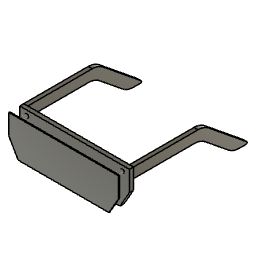
HyperShades mk.1 (Autodesk Fusion 360 design; units mm, degrees)
Autodesk Fusion 360 part; units mm, degrees
sketch "Sketch1" plane through (0, 0, 0) normal (0, 1, 0) x (1, 0, 0)
  line L0 (-69.215, 0) -> (69.215, 0)
  line L1 (-69.215, 0) -> (-69.215, 25.4)
  line L2 (69.215, 0) -> (69.215, 25.4)
  line L3 (69.215, 25.4) -> (57.1899, 46.228)
  line L4 (57.1899, 46.228) -> (-0.1294, 46.228)
  line L5 (-69.215, 25.4) -> (-57.1899, 46.228)
  line L6 (-57.1899, 46.228) -> (-0.1294, 46.228)
  dimension "d1" = 138.43
  dimension "d3" = 25.4
  dimension "d4" = 25.4
  dimension "d5" = 150
  dimension "d6" = 150
  dimension "d26" = 46.228
  constraint horizontal L0
  constraint coincident origin L0
  constraint perpendicular L0 L1
  constraint perpendicular L0 L2
  constraint coincident L0 origin
  constraint midpoint L0 origin
  constraint horizontal L4
  constraint horizontal L6
  measures "d1" distance of L0.start L0.end
  measures "d3" distance of L0.start L1.end
  measures "d4" distance of L0.end L2.end
  measures "d5" angle of L2 L3
  measures "d6" angle of L1 L5
  measures "d26" vertical distance of origin L4.end
extrude "Extrude1" add sketch "Sketch1" along normal blind 1.27 makes body 1
sketch "Sketch2" plane through (0, 1.27, 0) normal (0, 1, 0) x (-1, 0, 0)
  line L0 (69.215, 0) -> (-69.215, 0)
  line L1 (-69.215, 0) -> (-69.215, -25.4)
  line L2 (-69.215, -25.4) -> (-57.1899, -46.228)
  line L3 (-57.1899, -46.228) -> (57.1899, -46.228)
  line L4 (57.1899, -46.228) -> (69.215, -25.4)
  line L5 (69.215, -25.4) -> (69.215, 0)
  circle A0 centre (-60.325, -6.35) radius 2.286
  line L6 (-69.215, 0) -> (-60.325, 0) construction
  line L7 (-60.325, 0) -> (-60.325, -6.35) construction
  line L8 (-60.325, -6.35) -> (-69.215, -6.35) construction
  line L9 (-69.215, -6.35) -> (-69.215, 0) construction
  line L10 (69.215, 0) -> (60.325, 0) construction
  line L11 (60.325, 0) -> (60.325, -6.35) construction
  line L12 (60.325, -6.35) -> (69.215, -6.35) construction
  line L13 (69.215, -6.35) -> (69.215, 0) construction
  circle A1 centre (60.325, -6.35) radius 2.286
  line L14 (0, -46.228) -> (-12.7, -46.228) construction
  line L15 (-12.7, -46.228) -> (-12.7, -30.988) construction
  line L16 (-12.7, -30.988) -> (0, -30.988) construction
  line L17 (0, -30.988) -> (0, -46.228) construction
  line L18 (0, -46.228) -> (12.7, -46.228) construction
  line L19 (12.7, -46.228) -> (12.7, -30.988) construction
  line L20 (12.7, -30.988) -> (0, -30.988) construction
  line L21 (0, -30.988) -> (0, -46.228) construction
  circle A2 centre (-12.7, -30.988) radius 2.286
  circle A3 centre (12.7, -30.988) radius 2.286
  dimension "d10" = 4.572
  dimension "d11" = 8.89
  dimension "d12" = 6.35
  dimension "d23" = 8.89
  dimension "d24" = 6.35
  dimension "d25" = 4.572
  dimension "d27" = 12.7
  dimension "d28" = 15.24
  dimension "d29" = 12.7
  dimension "d30" = 15.24
  dimension "d31" = 4.572
  dimension "d32" = 4.572
  constraint horizontal L6
  constraint vertical L7
  constraint horizontal L8
  constraint vertical L9
  constraint coincident L0.end L1.start
  constraint coincident A0.centre L7.end
  constraint horizontal L10
  constraint vertical L11
  constraint horizontal L12
  constraint vertical L13
  constraint coincident L0.start L5.end
  constraint coincident L11.end L12.start
  constraint horizontal L14
  constraint vertical L15
  constraint horizontal L16
  constraint vertical L17
  constraint midpoint L3 L14.start
  constraint horizontal L18
  constraint vertical L19
  constraint horizontal L20
  constraint vertical L21
  constraint coincident L15.end L16.start
  constraint coincident L19.end L20.start
  measures "d10" diameter of A0
  measures "d11" distance of L0.end L6.end
  measures "d12" distance of L0.end L8.end
  measures "d23" distance of L0.start L10.end
  measures "d24" distance of L0.start L12.end
  measures "d25" diameter of A1
  measures "d27" distance of L14.start L14.end
  measures "d28" distance of L14.start L16.end
  measures "d29" distance of L14.start L18.end
  measures "d30" distance of L14.start L16.end
  measures "d31" diameter of A2
  measures "d32" diameter of A3
extrude "Extrude2" add sketch "Sketch2" along normal blind 12.7 separate body contours A0 | A1 | A2 | A3 makes body 2 at (58.0504, 9.7367, -6.5776) makes body 3 at (-62.5996, 9.7367, -6.5776) makes body 4 at (10.4254, 9.7367, -31.2156) makes body 5 at (-14.9746, 9.7367, -31.2156)
sketch "Sketch3" plane through (0, 13.97, 0) normal (0, 1, 0) x (-1, 0, 0)
  circle A0 centre (-60.325, -6.35) radius 2.286
  line L0 (69.215, 0) -> (-69.215, 0)
  line L1 (-69.215, 0) -> (-69.215, -25.4)
  line L2 (-69.215, -25.4) -> (-57.1899, -46.228)
  line L3 (-57.1899, -46.228) -> (57.1899, -46.228)
  line L4 (57.1899, -46.228) -> (69.215, -25.4)
  line L5 (69.215, -25.4) -> (69.215, 0)
  line L6 (-12.7, -46.228) -> (12.7, -46.228)
  line L7 (-12.7, -46.228) -> (-3.556, -22.4537)
  line L8 (3.556, -22.4537) -> (12.7, -46.228)
  arc A1 (3.556, -22.4537) -> (-3.556, -22.4537) centre (0, -23.8214) ccw
  circle A2 centre (-12.7, -30.988) radius 2.286
  circle A3 centre (12.7, -30.988) radius 2.286
  circle A4 centre (60.325, -6.35) radius 2.286
  point P0 (0, -46.228)
  point P1 (0, -13.208)
  dimension "d15" = 25.4
  dimension "d17" = 33.02
  dimension "d20" = 3.81
  constraint coincident L3 L6.start
  constraint parallel L3 L6
  constraint coincident L6 P0
  constraint midpoint L6 P0
  constraint vertical origin P0
  constraint vertical origin P1
  constraint coincident P1 L8
  constraint coincident P1 L7
  constraint tangent L8 A1
  constraint tangent L7 A1
  measures "d15" distance of L6.start L6.end
  measures "d17" vertical distance of L6.end P1
  measures "d20" radius of A1
extrude "Extrude4" add sketch "Sketch3" along normal blind 5.08 separate body contours L0 L1 L2 L3 L4 L5 L7 L8 A1 makes body 6
sketch "Sketch4" plane through (69.215, 0, 0) normal (1, 0, 0) x (0, 1, 0)
  line L0 (13.97, 0) -> (13.97, -25.4)
  line L1 (13.97, -25.4) -> (19.05, -25.4)
  line L2 (19.05, -25.4) -> (19.05, 0)
  line L3 (19.05, 0) -> (13.97, 0)
  line L4 (19.05, 0) -> (161.29, 0) construction
  line L5 (19.05, 0) -> (100.287, 0)
  line L6 (113.8983, -4.8311) -> (162.0907, -43.9722)
  line L7 (19.05, -12.7) -> (95.7793, -12.7)
  line L8 (109.3906, -17.5311) -> (138.7753, -41.3969)
  line L9 (152.3866, -46.228) -> (161.29, -46.228)
  arc A0 (138.7753, -41.3969) -> (152.3866, -46.228) centre (152.3866, -24.638) ccw
  arc A1 (161.29, -46.228) -> (162.0907, -43.9722) centre (161.29, -44.958) ccw
  arc A2 (109.3906, -17.5311) -> (95.7793, -12.7) centre (95.7793, -34.29) ccw
  arc A3 (113.8983, -4.8311) -> (100.287, 0) centre (100.287, -21.59) ccw
  point P0 (107.95, 0)
  point P1 (19.05, -46.228)
  dimension "d33" = 142.24
  dimension "d34" = 88.9
  dimension "d36" = 12.7
  dimension "d39" = 21.59
  dimension "d40" = 1.27
  dimension "d41" = 21.59
  dimension "d42" = 21.59
  constraint coincident L2.end L3.start
  constraint perpendicular L2 L4
  constraint perpendicular L2 L5
  constraint midpoint L2 L7.start
  constraint perpendicular L2 L7
  constraint parallel L6 L8
  constraint parallel L7 L9
  constraint tangent L8 A0
  constraint tangent L9 A0
  constraint tangent L6 A1
  constraint tangent L9 A1
  constraint tangent L7 A2
  constraint tangent L8 A2
  constraint coincident P0 L5
  constraint coincident P0 L6
  constraint tangent L5 A3
  constraint tangent L6 A3
  constraint horizontal P1 L9.start
  constraint vertical L4.end A1.centre
  measures "d33" distance of L2.end L4.end
  measures "d34" distance of L2.end P0
  measures "d36" distance of L6 L8
  measures "d39" radius of A0
  measures "d40" radius of A1
  measures "d41" radius of A2
  measures "d42" radius of A3
extrude "Extrude5" add sketch "Sketch4" against normal blind 5.08 separate body contours L2 L5 L6 L7 L8 L9 A0 A1 A2 A3 makes body 7
copy_body "CopyPasteBodies1" bodies 7 makes body 8
move_body "Move1" bodies 8 to x (1, 0, 0) y (0, 1, 0) z (0, 0, 1) at (-133.35, 0, 0)
equation "d21 = matThickness"
equation "d37 = -matThickness"
equation "matThickness = 0.2 in"
